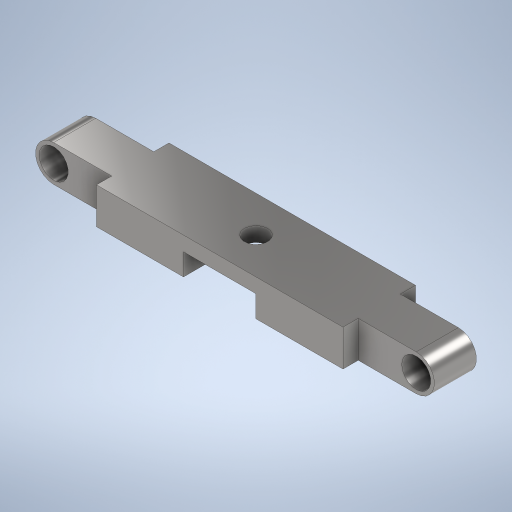
# Autodesk Inventor part: Przenośnik chwytaka
Saved by Autodesk Inventor 2024.1 (Build 281209000, 209)
## iProperties
Created: 2024-05-12
Part Number: Przenośnik chwytaka
Material: Stal, węglowa
Document SubType Name: Modeling
Designer: Krzysiu
Density: 7.85 g/cm^3
Appearance: Częściowo polerowany
Stock Number: 02
Mass: 14.2558 g
Surface Area: 16.375 cm^2
Volume: 1.81603 cm^3
Author: Krzysiu
Autodesk Inventor part; units mm, degrees
ref_plane "YZ Plane" through (0, 0, 0) normal (1, 0, 0) x (0, 1, 0)
ref_plane "XZ Plane" through (0, 0, 0) normal (0, 1, 0) x (-1, 0, 0)
ref_plane "XY Plane" through (0, 0, 0) normal (0, 0, 1) x (1, 0, 0)
sketch "Szkic1" plane through (0, 0, 0) normal (0, 0, 1) x (1, 0, 0)
  line L0 (0, 0) -> (-25, 0)
  line L1 (-25, 0) -> (-17.2354, -28.9778)
  line L2 (-25, 0) -> (5, 0) construction
  line L3 (-25, 0) -> (-34.8351, 36.7052)
  line L4 (-25, 0) -> (13, 0) construction
  line L5 (-34.8351, 36.7052) -> (-34.8351, 54.7052)
  line L6 (-34.8351, 54.7052) -> (0, 54.7052)
  line L7 (-34.8351, 54.7052) -> (-24.8351, 72.0257)
  line L8 (-34.8351, 54.7052) -> (-14.8351, 54.7052) construction
  line L9 (-34.8351, 54.7052) -> (-24.8351, 37.3847)
  line L10 (-34.8351, 54.7052) -> (-14.8351, 54.7052) construction
  circle A0 centre (-25, 0) radius 1.5
  line L11 (0, 0) -> (0, -12)
  line L12 (0, -12) -> (-25, -12)
  line L13 (-25, -12) -> (-17.2354, -28.9778)
  line L14 (-25, -12) -> (-45.5171, 32.862)
  line L15 (-45.5171, 32.862) -> (-48.5127, 50.611)
  line L16 (-45.5171, 32.862) -> (-27.5171, 32.862) construction
  line L17 (-48.5127, 50.611) -> (-35.7696, 35.1962)
  line L18 (-48.5127, 50.611) -> (-28.5127, 50.611) construction
  line L19 (-48.5127, 50.611) -> (-41.5347, 69.3542)
  line L20 (-48.5127, 50.611) -> (-28.5127, 50.611) construction
  circle A1 centre (-25, -12) radius 2.5
  line L21 (-17.2354, -28.9778) -> (2.5, -28.9778)
  circle A2 centre (-17.2354, -28.9778) radius 2.5
  line L22 (-19.7354, -28.9778) -> (-24.7354, -28.9778)
  line L23 (19.7354, -28.9778) -> (24.7354, -28.9778)
  circle A3 centre (17.2354, -28.9778) radius 2.5
  line L24 (25, -12) -> (17.2354, -28.9778)
  line L25 (17.2354, -28.9778) -> (2.5, -28.9778)
  line L26 (0, -12) -> (25, -12)
  line L27 (34.8351, 54.7052) -> (24.8351, 37.3847)
  line L28 (34.8351, 36.7052) -> (34.8351, 54.7052)
  line L29 (48.5127, 50.611) -> (35.7696, 35.1962)
  line L30 (45.5171, 32.862) -> (48.5127, 50.611)
  line L31 (45.5171, 32.862) -> (27.5171, 32.862) construction
  circle A4 centre (25, 0) radius 1.5
  line L32 (25, 0) -> (34.8351, 36.7052)
  circle A5 centre (25, -12) radius 2.5
  line L33 (25, -12) -> (45.5171, 32.862)
  line L34 (0, 0) -> (25, 0)
  line L35 (25, 0) -> (17.2354, -28.9778)
  line L36 (25, 0) -> (-5, 0) construction
  line L37 (25, 0) -> (-13, 0) construction
  line L38 (48.5127, 50.611) -> (28.5127, 50.611) construction
  line L39 (48.5127, 50.611) -> (28.5127, 50.611) construction
  line L40 (34.8351, 54.7052) -> (14.8351, 54.7052) construction
  line L41 (34.8351, 54.7052) -> (14.8351, 54.7052) construction
  line L42 (34.8351, 54.7052) -> (0, 54.7052)
  line L43 (48.5127, 50.611) -> (41.5347, 69.3542)
  line L44 (34.8351, 54.7052) -> (24.8351, 72.0257)
  line L45 (-17.2354, -31.4778) -> (-17.2354, -36.4778)
  line L46 (-17.2354, -36.4778) -> (2.5, -36.4778)
  line L47 (-17.2354, -36.4778) -> (-19.7354, -36.4778)
  line L48 (-24.7354, -28.9778) -> (-24.7354, -31.4778)
  line L49 (-17.2354, -26.4778) -> (-17.2354, -21.4778)
  line L50 (-17.2354, -21.4778) -> (-19.7354, -21.4778)
  line L51 (-24.7354, -26.4778) -> (-24.7354, -28.9778)
  line L52 (-17.2354, -21.4778) -> (2.5, -21.4778)
  line L53 (17.2354, -21.4778) -> (19.7354, -21.4778)
  line L54 (25, 0) -> (17.2354, -28.9778)
  line L55 (25, -12) -> (17.2354, -28.9778)
  line L56 (24.7354, -26.4778) -> (24.7354, -28.9778)
  line L57 (17.2354, -26.4778) -> (17.2354, -21.4778)
  line L58 (19.7354, -28.9778) -> (24.7354, -28.9778)
  circle A6 centre (17.2354, -28.9778) radius 2.5
  line L59 (24.7354, -28.9778) -> (24.7354, -31.4778)
  line L60 (17.2354, -36.4778) -> (19.7354, -36.4778)
  line L61 (17.2354, -31.4778) -> (17.2354, -36.4778)
  line L62 (17.2354, -28.9778) -> (-2.5, -28.9778)
  line L63 (17.2354, -36.4778) -> (-2.5, -36.4778)
  line L64 (17.2354, -21.4778) -> (-2.5, -21.4778)
  line L65 (-17.2354, -28.9778) -> (-2.5, -28.9778)
  arc A7 (-19.7354, -21.4778) -> (-24.7354, -26.4778) centre (-19.7354, -26.4778) ccw
  arc A8 (-24.7354, -31.4778) -> (-19.7354, -36.4778) centre (-19.7354, -31.4778) ccw
  arc A9 (24.7354, -26.4778) -> (19.7354, -21.4778) centre (19.7354, -26.4778) ccw
  arc A10 (19.7354, -36.4778) -> (24.7354, -31.4778) centre (19.7354, -31.4778) ccw
  line L66 (25, -14.5) -> (0, -14.5)
  line L67 (0, -14.5) -> (-25, -14.5)
  line L68 (-25, -9.5) -> (0, -9.5)
  line L69 (25, -9.5) -> (0, -9.5)
  point P0 (0, 0)
  point P1 (0, 0)
  point P2 (2.5, 0)
  point P3 (-24.7354, -36.4778)
  point P4 (-24.7354, -21.4778)
  point P5 (24.7354, -21.4778)
  point P6 (24.7354, -36.4778)
  dimension "d0" = 25
  dimension "d1" = 30
  dimension "d2" = 75
  dimension "d3" = 38
  dimension "d4" = 105
  dimension "d5" = 18
  dimension "d6" = 20
  dimension "d7" = 60
  dimension "d8" = 20
  dimension "d9" = 60
  dimension "d10" = 3
  dimension "d11" = 12
  dimension "d12" = 25
  dimension "d13" = 49.331
  dimension "d14" = 18
  dimension "d15" = 99.58
  dimension "d16" = 20
  dimension "d17" = 50.42
  dimension "d18" = 20
  dimension "d19" = 69.58
  dimension "d20" = 5
  dimension "d21" = 5
  dimension "d22" = 5
  dimension "d23" = 5
  dimension "d24" = 5
  dimension "d25" = 5
  dimension "d26" = 5
  dimension "d27" = 5
  dimension "d28" = 5
  constraints: 140 end point, 37 symmetric about line, 18 point on circle, 15 point on line, 13 horizontal, 11 tangent, 10 centre point, 10 coincident, 9 perpendicular, 7 equal length, 2 vertical, 1 horizontal alignment, 6 other
  measures "d0" distance of L0.start L0.end
  measures "d1" distance of L0.end L1.end
  measures "d2" angle of L1 L2
  measures "d3" distance of L0.end L3.end
  measures "d4" angle of L4 L3
  measures "d5" distance of L3.end L5.end
  measures "d6" distance of L5.end L7.end
  measures "d7" angle of L8 L7
  measures "d8" distance of L5.end L9.end
  measures "d9" angle of L9 L10
  measures "d10" diameter of A0
  measures "d11" distance of L0.start L11.end
  measures "d12" distance of L11.end L12.end
  measures "d13" distance of L12.end L14.end
  measures "d14" distance of L14.end L15.end
  measures "d15" angle of L16 L15
  measures "d16" distance of L15.end L17.end
  measures "d17" angle of L17 L18
  measures "d18" distance of L15.end L19.end
  measures "d19" angle of L20 L19
  measures "d20" diameter of A1
  measures "d21" diameter of A2
  measures "d22" distance of L22.start L22.end
  measures "d23" distance of L45.start L45.end
  measures "d24" distance of L49.start L49.end
  measures "d25" radius of A7
  measures "d26" radius of A8
  measures "d27" radius of A9
  measures "d28" radius of A10
extrude "Wyciągnięcie proste1" add sketch "Szkic1" along normal mid plane 30 contours A1 L12 L14 | A5 L33 L26 | A1 L13 L12 | L26 L24 A5 | L14 L13 A1 | A5 L24 L33
extrude "Wyciągnięcie proste2" add sketch "Szkic1" along normal mid plane 10 contours L69 L35 L26 L11 | L11 L12 L1 L68 | L26 L35 L66 L67 L1 L12 | L1 L12 A1 L68 | L69 A5 L26 L35 | L1 L67 L13 A1 L12 | L26 A5 L24 L66 L35 | L67 A1 L13 | A5 L66 L24
sketch "Szkic2" plane through (-25, -12, 15) normal (0, 0, 1) x (1, 0, 0)
  circle A0 centre (0, 0) radius 2.5
  point P0 (25, 12)
  constraints: 1 centre point
extrude "Wyciągnięcie proste3" cut sketch "Szkic2" against normal blind 10
sketch "Szkic3" plane through (-25, -12, -15) normal (0, 0, -1) x (-1, 0, 0)
  circle A0 centre (0, 0) radius 2.5
  point P0 (-25, 12)
  constraints: 1 centre point
extrude "Wyciągnięcie proste4" cut sketch "Szkic3" against normal blind 10
sketch "Szkic4" plane through (25, -12, 15) normal (0, 0, 1) x (1, 0, 0)
  circle A0 centre (0, 0) radius 2.5
  point P0 (-25, 12)
  constraints: 1 centre point
extrude "Wyciągnięcie proste5" cut sketch "Szkic4" against normal blind 10
sketch "Szkic5" plane through (25, -12, -15) normal (0, 0, -1) x (-1, 0, 0)
  circle A0 centre (0, 0) radius 2.5
  point P0 (25, 12)
  constraints: 1 centre point
extrude "Wyciągnięcie proste6" cut sketch "Szkic5" against normal blind 10
sketch "Szkic6" plane through (0, 0, 5) normal (0, 0, 1) x (1, 0, 0)
  arc A0 (-25, -9.5) -> (-25, -14.5) centre (-25, -12) ccw projected
  arc A1 (25, -14.5) -> (25, -9.5) centre (25, -12) ccw projected
  circle A2 centre (-25, -12) radius 2
  circle A3 centre (25, -12) radius 2
  point P0 (0, 0)
  dimension "d41" = 4
  dimension "d42" = 4
  constraints: 2 centre point, 2 coincident
  measures "d41" diameter of A2
  measures "d42" diameter of A3
extrude "Wyciągnięcie proste7" cut sketch "Szkic6" against normal blind 10
sketch "Szkic7" plane through (-25, -14.5, 5) normal (0, -1, 0) x (1, 0, 0)
  circle A0 centre (25, -5) radius 1.6
  dimension "d45" = 3.2
  constraints: 1 centre point, 1 coincident
  measures "d45" diameter of A0
extrude "Wyciągnięcie proste8" cut sketch "Szkic7" against normal blind 10
sketch "Szkic8" plane through (-25, -14.5, 5) normal (0, -1, 0) x (1, 0, 0)
  line L0 (25, -5) -> (25, -10)
  line L1 (0, -10) -> (50, -10) projected
  line L2 (25, -5) -> (25, 0)
  line L3 (50, 0) -> (0, 0) projected
  line L4 (25, -10) -> (30, -10)
  line L5 (30, -10) -> (30, 0)
  line L6 (30, 0) -> (25, 0)
  line L7 (24.8317, 0) -> (19.8317, 0)
  line L8 (19.8317, 0) -> (19.8317, -10)
  line L9 (19.8317, -10) -> (25, -10)
  dimension "d48" = 5
  dimension "d49" = 5
  constraints: 16 end point, 5 perpendicular, 3 point on line, 2 midpoint
  measures "d48" distance of L0.end L4.end
  measures "d49" distance of L7.start L7.end
extrude "Wyciągnięcie proste9" cut sketch "Szkic8" against normal blind 2
sketch "Szkic9" plane through (-25, -12.5, 5) normal (0, -1, 0) x (1, 0, 0)
  line L0 (19.8317, -10) -> (19.8317, 0) projected
  line L1 (19.8317, 0) -> (19.8317, -10)
  line L2 (0, -10) -> (50, -10) projected
  line L3 (19.8317, -10) -> (29.8317, -10)
  line L4 (29.8317, 0) -> (19.8317, 0)
  line L5 (30, 0) -> (50, 0) projected
  line L6 (30, 0) -> (30, -10)
  line L7 (30, -10) -> (20, -10)
  line L8 (20, -10) -> (20, 0)
  point P0 (25, -5)
  dimension "d52" = 10
  dimension "d53" = 10
  constraints: 12 end point, 4 point on line, 3 perpendicular, 1 vertical
  measures "d52" distance of L1.end L3.end
  measures "d53" distance of L6.end L7.end
extrude "Wyciągnięcie proste10" add sketch "Szkic9" along normal blind 2
sketch "Szkic10" plane through (-25, -12.5, 5) normal (0, -1, 0) x (1, 0, 0)
  line L0 (0, 0) -> (20, 0) projected
  line L1 (20, 0) -> (30, 0)
  line L2 (50, 0) -> (0, 0) projected
  line L3 (30, 0) -> (30, -10.0332)
  line L4 (30, 0) -> (30, -10)
  line L5 (30, -10) -> (20, -10)
  line L6 (20, -10) -> (20, 0)
  point P0 (25, -5)
  dimension "d56" = 10
  dimension "d57" = 10
  dimension "d58" = 10
  constraints: 10 end point, 2 perpendicular, 2 point on line
  measures "d56" distance of L0.end L1.end
  measures "d57" distance of L1.end L4.end
  measures "d58" distance of L4.end L5.end
extrude "Wyciągnięcie proste11" cut sketch "Szkic10" against normal blind 1
sketch "Szkic11" plane through (0, 0, 5) normal (0, 0, 1) x (1, 0, 0)
  arc A0 (-25, -9.5) -> (-25, -14.5) centre (-25, -12) ccw projected
  line L0 (-25, -9.5) -> (-17, -9.5)
  line L1 (-25, -9.5) -> (25, -9.5) projected
  line L2 (-25, -14.5) -> (-5, -14.5) projected
  line L3 (5, -14.5) -> (25, -14.5) projected
  line L4 (-25, -14.5) -> (-17, -14.5)
  line L5 (-17, -14.5) -> (-17, -9.5)
  arc A1 (-25, -9.5) -> (-25, -14.5) centre (-25, -12) ccw projected
  arc A2 (-25, -9.5) -> (-25, -14.5) centre (-25, -12) ccw
  line L6 (-17, -14.5) -> (-25, -14.5)
  arc A3 (25, -14.5) -> (25, -9.5) centre (25, -12) ccw
  line L7 (25, -9.5) -> (17, -9.5)
  line L8 (17, -9.5) -> (17, -14.5)
  line L9 (25, -14.5) -> (17, -14.5)
  point P0 (0, 0)
  dimension "d61" = 8
  dimension "d62" = 8
  dimension "d63" = 8
  constraints: 17 end point, 4 point on circle, 4 point on line, 2 centre point, 2 perpendicular, 1 coincident, 1 horizontal
  measures "d61" distance of L0.start L0.end
  measures "d62" distance of L2.start L4.end
  measures "d63" distance of L1.end L7.end
extrude "Wyciągnięcie proste12" cut sketch "Szkic11" against normal blind 2.1 from surface at 0
sketch "Szkic12" plane through (0, 0, -5) normal (0, 0, -1) x (-1, 0, 0)
  circle A0 centre (-25, -12) radius 2 projected
  arc A1 (-25, -9.5) -> (-25, -14.5) centre (-25, -12) ccw
  circle A2 centre (25, -12) radius 2 projected
  line L0 (17, -9.5) -> (25, -9.5) projected
  arc A3 (25, -14.5) -> (25, -9.5) centre (25, -12) ccw
  line L1 (-25, -9.5) -> (-17, -9.5)
  line L2 (25, -9.5) -> (-25, -9.5) projected
  line L3 (-17, -9.5) -> (-17, -14.5)
  line L4 (-17, -14.5) -> (-25, -14.5)
  line L5 (25, -14.5) -> (17, -14.5)
  line L6 (17, -14.5) -> (17, -9.5)
  line L7 (25, -9.5) -> (17, -9.5)
  point P0 (0, 0)
  dimension "d66" = 8
  dimension "d67" = 8
  constraints: 13 end point, 4 point on circle, 3 point on line, 2 centre point, 2 coincident, 2 perpendicular, 2 tangent, 1 collinear
  measures "d66" distance of L1.start L1.end
  measures "d67" distance of L5.start L5.end
extrude "Wyciągnięcie proste13" cut sketch "Szkic12" against normal blind 2.1
